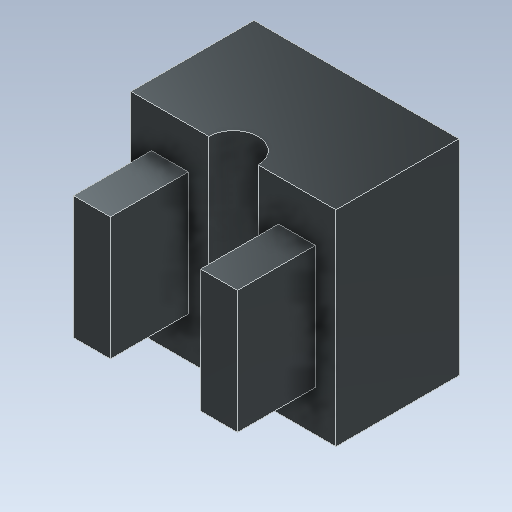
# Autodesk Inventor part: laser top
Saved by Autodesk Inventor 2021 (Build 250183000, 183)
## iProperties
Created: 2021-06-12
Part Number: laser top
Material: Iron, Cast
Document SubType Name: Modeling
Designer: user
Density: 7.15 g/cm^3
Appearance: Iron Gray
Author: user
Autodesk Inventor part; units mm, degrees
ref_plane "YZ Plane" through (0, 0, 0) normal (1, 0, 0) x (0, 1, 0)
ref_plane "XZ Plane" through (0, 0, 0) normal (0, 1, 0) x (-1, 0, 0)
ref_plane "XY Plane" through (0, 0, 0) normal (0, 0, 1) x (1, 0, 0)
sketch "Sketch1" plane through (0, 0, 0) normal (0, 0, 1) x (1, 0, 0)
  line L0 (-23.6135, 32.149) -> (26.3865, 32.149)
  line L1 (26.3865, 32.149) -> (26.3865, -17.851)
  line L2 (26.3865, -17.851) -> (-23.6135, -17.851)
  line L3 (-23.6135, -17.851) -> (-23.6135, 32.149)
  point P0 (0, 0)
  dimension "d0" = 50
  dimension "d1" = 50
  constraints: 8 end point, 2 parallel, 1 horizontal, 1 perpendicular
  measures "d0" distance of L0.start L0.end
  measures "d1" distance of L2.end L0.start
extrude "Extrusion1" add sketch "Sketch1" along normal blind 30
sketch "Sketch2" plane through (0, 0, 30) normal (0, 0, 1) x (1, 0, 0)
  line L0 (12.3865, 22.149) -> (21.3865, 22.149)
  line L1 (21.3865, 22.149) -> (21.3865, -7.851)
  line L2 (21.3865, -7.851) -> (12.3865, -7.851)
  line L3 (12.3865, -7.851) -> (12.3865, 22.149)
  line L4 (-18.6135, 22.149) -> (-9.6135, 22.149)
  line L5 (-9.6135, 22.149) -> (-9.6135, -7.851)
  line L6 (-9.6135, -7.851) -> (-18.6135, -7.851)
  line L7 (-18.6135, -7.851) -> (-18.6135, 22.149)
  line L8 (26.3865, 32.149) -> (-23.6135, 32.149) projected
  line L9 (-23.6135, -17.851) -> (26.3865, -17.851) projected
  line L10 (26.3865, -17.851) -> (26.3865, 32.149) projected
  line L11 (-23.6135, 32.149) -> (-23.6135, -17.851) projected
  point P0 (0, 0)
  dimension "d4" = 10
  dimension "d5" = 10
  dimension "d6" = 5
  dimension "d7" = 5
  dimension "d11" = 9
  dimension "d12" = 9
  constraints: 16 end point, 4 parallel, 2 horizontal, 2 perpendicular, 2 point on line
  measures "d4" distance between parallel lines of L8 L4
  measures "d5" distance between parallel lines of L9 L6
  measures "d6" distance between parallel lines of L10 L1
  measures "d7" distance between parallel lines of L11 L7
  measures "d11" distance of L0.start L0.end
  measures "d12" distance of L4.start L4.end
sketch "Sketch3" plane through (-23.6135, -17.851, 0) normal (0, -1, 0) x (1, 0, 0)
  line L0 (0, 30) -> (50, 30) projected
  circle A0 centre (25, 30) radius 6
  point P0 (23.6135, 0)
  dimension "d8" = 12
  dimension "d13" = 25
  constraints: 1 centre point, 1 midpoint
  measures "d8" diameter of A0
  measures "d13" distance of L0.end A0.centre
extrude "Extrusion2" cut sketch "Sketch3" against normal blind 50
extrude "Extrusion3" add sketch "Sketch2" along normal blind 19 contours L0 L1 L2 L3 | L4 L5 L6 L7
equation "\"d1\" = d0"
body "Solid1"
